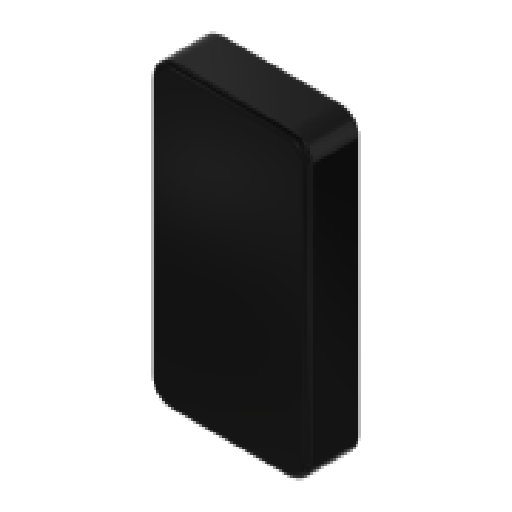
# Autodesk Inventor part: powerbank
Saved by Autodesk Inventor 2026.1 (Build 301233020, 233B)
## iProperties
Created: 2026-02-19
Part Number: powerbank
Material: PC/ABS Plastic
Document SubType Name: Modeling
Designer: samuel
Density: 1.1 g/cm^3
Appearance: Smooth - Black
Author: samuel
Autodesk Inventor part; units mm, degrees
ref_plane "YZ Plane" through (0, 0, 0) normal (1, 0, 0) x (0, 1, 0)
ref_plane "XZ Plane" through (0, 0, 0) normal (0, 1, 0) x (-1, 0, 0)
ref_plane "XY Plane" through (0, 0, 0) normal (0, 0, 1) x (1, 0, 0)
sketch "Sketch1" plane through (0, 0, 0) normal (0, 0, 1) x (1, 0, 0)
  line L0 (-35.5, -67) -> (35.5, -67)
  line L1 (35.5, -67) -> (35.5, 67)
  line L2 (35.5, 67) -> (-35.5, 67)
  line L3 (-35.5, 67) -> (-35.5, -67)
  line L4 (-35.5, -67) -> (35.5, 67) construction
  line L5 (35.5, -67) -> (-35.5, 67) construction
  point P0 (0, 0)
  dimension "d0" = 71
  dimension "d1" = 134
  constraints: 12 end point, 2 midpoint, 2 parallel, 1 horizontal, 1 perpendicular
  measures "d0" distance of L2.end L1.end
  measures "d1" distance of L1.end L0.end
extrude "Extrusion1" add sketch "Sketch1" along normal blind 25
fillet "Fillet1" radius 10 4 edges at (-35.5, 67, 12.5) (35.5, 67, 12.5) (-35.5, -67, 12.5) (35.5, -67, 12.5)
fillet "Fillet2" radius 3 16 edges at (-32.5711, -64.0711, 0) (0, -67, 0) (32.5711, -64.0711, 0) (35.5, 0, 0) (32.5711, 64.0711, 0) (0, 67, 0) (-32.5711, 64.0711, 0) (-35.5, 0, 0) (0, 67, 25) (32.5711, 64.0711, 25) (35.5, 0, 25) (32.5711, -64.0711, 25) (0, -67, 25) (-32.5711, -64.0711, 25) (-35.5, 0, 25) (-32.5711, 64.0711, 25)
body "Solid1"
